Autodesk Fusion 360 part; units mm, degrees
note: some values were not read from the file. Chosen so that the rebuilt part matches the saved one: which bodies a step acts on. Set by a fixed rule: which sketch regions a step uses.
(part 3 of 6)
  spline S61 degree 5 poles (-154.2027, 37.7428) (-154.1706, 37.7034) (-154.1065, 37.6251) (-154.0104, 37.5085) (-153.8824, 37.355) (-153.7229, 37.1664) (-153.5638, 36.9811) (-153.4052, 36.7992) (-153.247, 36.6207) (-153.0893, 36.4456) (-152.9323, 36.2741) (-152.776, 36.106) (-152.6205, 35.9416) (-152.4659, 35.7807) (-152.3123, 35.6233) (-152.1597, 35.4696) (-152.0083, 35.3195) (-151.858, 35.173) (-151.709, 35.0302) (-151.5613, 34.8912) (-151.4153, 34.756) (-151.2709, 34.6246) (-151.1283, 34.4971) (-150.9877, 34.3737) (-150.8492, 34.2541) (-150.7127, 34.1386) (-150.6052, 34.0492) (-150.5255, 33.9839) (-150.4728, 33.9412) (-150.4466, 33.92) knots 0 0 0 0 0 0 0.04 0.08 0.12 0.16 0.2 0.24 0.28 0.32 0.36 0.4 0.44 0.48 0.52 0.56 0.6 0.64 0.68 0.72 0.76 0.8 0.84 0.88 0.92 0.96 1 1 1 1 1 1
  arc A61 (-156.6092, 32.582) -> (-150.4466, 33.92) centre (-153.9133, 35.0261) ccw
  spline S62 degree 5 poles (-156.6092, 32.582) (-156.5585, 32.5827) (-156.4572, 32.5839) (-156.3061, 32.5852) (-156.1063, 32.5859) (-155.8593, 32.585) (-155.6151, 32.5822) (-155.3737, 32.5776) (-155.1353, 32.5711) (-154.8999, 32.5629) (-154.6675, 32.5529) (-154.4384, 32.5411) (-154.2124, 32.5278) (-153.9898, 32.5128) (-153.7705, 32.4962) (-153.5547, 32.4782) (-153.3423, 32.4586) (-153.1335, 32.4376) (-152.9283, 32.4153) (-152.7269, 32.3915) (-152.5294, 32.3666) (-152.336, 32.3404) (-152.1468, 32.3131) (-151.9618, 32.2848) (-151.7812, 32.2555) (-151.6049, 32.2253) (-151.4674, 32.2003) (-151.3661, 32.1812) (-151.2995, 32.1683) (-151.2664, 32.1618) knots 0 0 0 0 0 0 0.04 0.08 0.12 0.16 0.2 0.24 0.28 0.32 0.36 0.4 0.44 0.48 0.52 0.56 0.6 0.64 0.68 0.72 0.76 0.8 0.84 0.88 0.92 0.96 1 1 1 1 1 1
  arc A62 (-151.2664, 32.1618) -> (-157.2099, 31.1319) centre (-153.9947, 30.2418) ccw
  spline S63 degree 5 poles (-157.2099, 31.1319) (-157.1745, 31.0955) (-157.1037, 31.0231) (-156.9978, 30.9153) (-156.857, 30.7736) (-156.6816, 30.5996) (-156.507, 30.4288) (-156.3331, 30.2614) (-156.1599, 30.0974) (-155.9876, 29.9368) (-155.8163, 29.7796) (-155.6459, 29.6258) (-155.4767, 29.4755) (-155.3087, 29.3287) (-155.1419, 29.1853) (-154.9765, 29.0455) (-154.8125, 28.9091) (-154.6501, 28.7763) (-154.4892, 28.6471) (-154.33, 28.5214) (-154.1727, 28.3994) (-154.0174, 28.2812) (-153.8643, 28.1666) (-153.7135, 28.0559) (-153.5651, 27.9489) (-153.419, 27.8456) (-153.3042, 27.766) (-153.2191, 27.7079) (-153.1628, 27.6699) (-153.1348, 27.6511) knots 0 0 0 0 0 0 0.04 0.08 0.12 0.16 0.2 0.24 0.28 0.32 0.36 0.4 0.44 0.48 0.52 0.56 0.6 0.64 0.68 0.72 0.76 0.8 0.84 0.88 0.92 0.96 1 1 1 1 1 1
  arc A63 (-159.1574, 25.7811) -> (-153.1348, 27.6511) centre (-156.6848, 28.4509) ccw
  spline S64 degree 5 poles (-159.1574, 25.7811) (-159.1069, 25.7862) (-159.0061, 25.7963) (-158.8557, 25.8107) (-158.6567, 25.8288) (-158.4106, 25.8494) (-158.167, 25.8679) (-157.9262, 25.8843) (-157.6881, 25.8987) (-157.4529, 25.911) (-157.2206, 25.9213) (-156.9913, 25.9296) (-156.765, 25.9359) (-156.5419, 25.9404) (-156.322, 25.943) (-156.1054, 25.9439) (-155.8922, 25.9429) (-155.6823, 25.9402) (-155.476, 25.9358) (-155.2733, 25.9297) (-155.0744, 25.922) (-154.8794, 25.9128) (-154.6885, 25.9021) (-154.5018, 25.8901) (-154.3193, 25.8766) (-154.1411, 25.8619) (-154.0019, 25.849) (-153.8994, 25.8388) (-153.8319, 25.8318) (-153.7983, 25.8282) knots 0 0 0 0 0 0 0.04 0.08 0.12 0.16 0.2 0.24 0.28 0.32 0.36 0.4 0.44 0.48 0.52 0.56 0.6 0.64 0.68 0.72 0.76 0.8 0.84 0.88 0.92 0.96 1 1 1 1 1 1
  arc A64 (-153.7983, 25.8282) -> (-159.6294, 24.2842) centre (-156.3488, 23.6776) ccw
  spline S65 degree 5 poles (-159.6294, 24.2842) (-159.591, 24.251) (-159.5142, 24.185) (-159.3993, 24.0869) (-159.2466, 23.9579) (-159.0568, 23.7999) (-158.8679, 23.645) (-158.6801, 23.4934) (-158.4933, 23.3451) (-158.3077, 23.2001) (-158.1232, 23.0584) (-157.9401, 22.9201) (-157.7584, 22.7851) (-157.5783, 22.6535) (-157.3997, 22.5252) (-157.2227, 22.4003) (-157.0475, 22.2788) (-156.874, 22.1606) (-156.7025, 22.0459) (-156.533, 21.9346) (-156.3656, 21.8268) (-156.2006, 21.7225) (-156.0381, 21.6218) (-155.8782, 21.5246) (-155.721, 21.4309) (-155.5666, 21.3408) (-155.4452, 21.2715) (-155.3553, 21.221) (-155.296, 21.1881) (-155.2665, 21.1718) knots 0 0 0 0 0 0 0.04 0.08 0.12 0.16 0.2 0.24 0.28 0.32 0.36 0.4 0.44 0.48 0.52 0.56 0.6 0.64 0.68 0.72 0.76 0.8 0.84 0.88 0.92 0.96 1 1 1 1 1 1
  arc A65 (-161.1032, 18.784) -> (-155.2665, 21.1718) centre (-158.8726, 21.6591) ccw
  spline S66 degree 5 poles (-161.1032, 18.784) (-161.0533, 18.7935) (-160.9538, 18.8123) (-160.8052, 18.8398) (-160.6086, 18.8751) (-160.3651, 18.9171) (-160.1241, 18.9568) (-159.8857, 18.9941) (-159.6497, 19.0292) (-159.4165, 19.062) (-159.1859, 19.0924) (-158.9582, 19.1207) (-158.7334, 19.1467) (-158.5115, 19.1706) (-158.2927, 19.1924) (-158.077, 19.2121) (-157.8644, 19.2297) (-157.6552, 19.2453) (-157.4492, 19.2589) (-157.2468, 19.2705) (-157.048, 19.2802) (-156.8529, 19.2881) (-156.6618, 19.2941) (-156.4747, 19.2983) (-156.2918, 19.3008) (-156.113, 19.3016) (-155.9732, 19.301) (-155.8702, 19.2997) (-155.8023, 19.2986) (-155.7686, 19.2979) knots 0 0 0 0 0 0 0.04 0.08 0.12 0.16 0.2 0.24 0.28 0.32 0.36 0.4 0.44 0.48 0.52 0.56 0.6 0.64 0.68 0.72 0.76 0.8 0.84 0.88 0.92 0.96 1 1 1 1 1 1
  arc A66 (-155.7686, 19.2979) -> (-161.4429, 17.2516) centre (-158.1219, 16.9333) ccw
  spline S67 degree 5 poles (-161.4429, 17.2516) (-161.4017, 17.2219) (-161.3194, 17.1628) (-161.1964, 17.0751) (-161.0331, 16.96) (-160.8302, 16.8191) (-160.6286, 16.6813) (-160.4283, 16.5466) (-160.2293, 16.4151) (-160.0317, 16.2868) (-159.8356, 16.1618) (-159.6412, 16.0399) (-159.4484, 15.9213) (-159.2574, 15.8059) (-159.0683, 15.6937) (-158.8812, 15.5847) (-158.696, 15.4789) (-158.5129, 15.3763) (-158.332, 15.277) (-158.1534, 15.1809) (-157.9773, 15.088) (-157.8039, 14.9985) (-157.6332, 14.9123) (-157.4655, 14.8294) (-157.3007, 14.7498) (-157.139, 14.6735) (-157.012, 14.615) (-156.9181, 14.5726) (-156.8561, 14.545) (-156.8253, 14.5313) knots 0 0 0 0 0 0 0.04 0.08 0.12 0.16 0.2 0.24 0.28 0.32 0.36 0.4 0.44 0.48 0.52 0.56 0.6 0.64 0.68 0.72 0.76 0.8 0.84 0.88 0.92 0.96 1 1 1 1 1 1
  arc A67 (-162.4317, 11.6439) -> (-156.8253, 14.5313) centre (-160.4602, 14.7025) ccw
  spline S68 degree 5 poles (-162.4317, 11.6439) (-162.3828, 11.6577) (-162.2853, 11.6851) (-162.1397, 11.7255) (-161.9469, 11.7778) (-161.708, 11.8408) (-161.4714, 11.9013) (-161.2371, 11.9594) (-161.0051, 12.0149) (-160.7756, 12.0678) (-160.5486, 12.1183) (-160.3242, 12.1663) (-160.1025, 12.2118) (-159.8836, 12.255) (-159.6675, 12.2957) (-159.4543, 12.3341) (-159.2441, 12.3702) (-159.037, 12.404) (-158.8331, 12.4355) (-158.6324, 12.4647) (-158.4351, 12.4917) (-158.2415, 12.5165) (-158.0517, 12.5391) (-157.8657, 12.5596) (-157.6836, 12.5781) (-157.5056, 12.5945) (-157.3663, 12.606) (-157.2635, 12.6138) (-157.1958, 12.6186) (-157.1622, 12.6208) knots 0 0 0 0 0 0 0.04 0.08 0.12 0.16 0.2 0.24 0.28 0.32 0.36 0.4 0.44 0.48 0.52 0.56 0.6 0.64 0.68 0.72 0.76 0.8 0.84 0.88 0.92 0.96 1 1 1 1 1 1
  arc A68 (-157.1622, 12.6208) -> (-162.6366, 10.0878) centre (-159.3005, 10.0601) ccw
  spline S69 degree 5 poles (-162.6366, 10.0878) (-162.5929, 10.0618) (-162.5058, 10.0101) (-162.3757, 9.9334) (-162.2029, 9.8329) (-161.9885, 9.7102) (-161.7757, 9.5905) (-161.5643, 9.4739) (-161.3546, 9.3602) (-161.1466, 9.2496) (-160.9404, 9.1422) (-160.7361, 9.0377) (-160.5337, 8.9363) (-160.3334, 8.838) (-160.1352, 8.7427) (-159.9393, 8.6504) (-159.7456, 8.5612) (-159.5543, 8.4749) (-159.3654, 8.3917) (-159.1791, 8.3116) (-158.9956, 8.2345) (-158.815, 8.1604) (-158.6375, 8.0894) (-158.4631, 8.0214) (-158.2921, 7.9565) (-158.1243, 7.8946) (-157.9927, 7.8474) (-157.8955, 7.8133) (-157.8314, 7.7912) (-157.7994, 7.7802) knots 0 0 0 0 0 0 0.04 0.08 0.12 0.16 0.2 0.24 0.28 0.32 0.36 0.4 0.44 0.48 0.52 0.56 0.6 0.64 0.68 0.72 0.76 0.8 0.84 0.88 0.92 0.96 1 1 1 1 1 1
  arc A69 (-163.1328, 4.4152) -> (-157.7994, 7.7802) centre (-161.4354, 7.634) ccw
  spline S70 degree 5 poles (-163.1328, 4.4152) (-163.0854, 4.4332) (-162.9906, 4.469) (-162.8491, 4.5219) (-162.6616, 4.5909) (-162.4291, 4.6744) (-162.1987, 4.7554) (-161.9703, 4.8336) (-161.7441, 4.9091) (-161.52, 4.9818) (-161.2983, 5.0519) (-161.0789, 5.1193) (-160.862, 5.184) (-160.6477, 5.246) (-160.436, 5.3055) (-160.227, 5.3623) (-160.0207, 5.4166) (-159.8173, 5.4683) (-159.6169, 5.5174) (-159.4195, 5.564) (-159.2254, 5.6081) (-159.0347, 5.6497) (-158.8475, 5.6888) (-158.664, 5.7254) (-158.4843, 5.7596) (-158.3083, 5.7915) (-158.1705, 5.8151) (-158.0689, 5.8318) (-158.0018, 5.8425) (-157.9685, 5.8477) knots 0 0 0 0 0 0 0.04 0.08 0.12 0.16 0.2 0.24 0.28 0.32 0.36 0.4 0.44 0.48 0.52 0.56 0.6 0.64 0.68 0.72 0.76 0.8 0.84 0.88 0.92 0.96 1 1 1 1 1 1
  arc A70 (-157.9685, 5.8477) -> (-163.2013, 2.8471) centre (-159.8755, 3.1103) ccw
  spline S71 degree 5 poles (-163.2013, 2.8471) (-163.1556, 2.825) (-163.0643, 2.7811) (-162.9279, 2.7161) (-162.7471, 2.631) (-162.5228, 2.5275) (-162.3003, 2.4268) (-162.0797, 2.329) (-161.8609, 2.2341) (-161.644, 2.1421) (-161.4292, 2.0529) (-161.2166, 1.9667) (-161.0061, 1.8834) (-160.798, 1.8029) (-160.5923, 1.7252) (-160.389, 1.6503) (-160.1883, 1.5783) (-159.9902, 1.5091) (-159.7948, 1.4426) (-159.6022, 1.379) (-159.4127, 1.3182) (-159.2263, 1.2602) (-159.0433, 1.2049) (-158.8637, 1.1524) (-158.6876, 1.1026) (-158.5151, 1.0555) (-158.3799, 1.02) (-158.2801, 0.9945) (-158.2142, 0.9781) (-158.1815, 0.97) knots 0 0 0 0 0 0 0.04 0.08 0.12 0.16 0.2 0.24 0.28 0.32 0.36 0.4 0.44 0.48 0.52 0.56 0.6 0.64 0.68 0.72 0.76 0.8 0.84 0.88 0.92 0.96 1 1 1 1 1 1
  arc A71 (-163.2013, -2.8471) -> (-158.1815, 0.97) centre (-161.7909, 0.5074) ccw
  spline S72 degree 5 poles (-163.2013, -2.8471) (-163.1556, -2.825) (-163.0643, -2.7811) (-162.9279, -2.7161) (-162.7471, -2.631) (-162.5228, -2.5275) (-162.3003, -2.4268) (-162.0797, -2.329) (-161.8609, -2.2341) (-161.644, -2.1421) (-161.4292, -2.0529) (-161.2166, -1.9667) (-161.0061, -1.8834) (-160.798, -1.8029) (-160.5923, -1.7252) (-160.389, -1.6503) (-160.1883, -1.5783) (-159.9902, -1.5091) (-159.7948, -1.4426) (-159.6022, -1.379) (-159.4127, -1.3182) (-159.2263, -1.2602) (-159.0433, -1.2049) (-158.8637, -1.1524) (-158.6876, -1.1026) (-158.5151, -1.0555) (-158.3799, -1.02) (-158.2801, -0.9945) (-158.2142, -0.9781) (-158.1815, -0.97) knots 0 0 0 0 0 0 0.04 0.08 0.12 0.16 0.2 0.24 0.28 0.32 0.36 0.4 0.44 0.48 0.52 0.56 0.6 0.64 0.68 0.72 0.76 0.8 0.84 0.88 0.92 0.96 1 1 1 1 1 1
  arc A72 (-158.1815, -0.97) -> (-163.1328, -4.4152) centre (-159.8427, -3.8631) ccw
  spline S73 degree 5 poles (-163.1328, -4.4152) (-163.0854, -4.4332) (-162.9906, -4.469) (-162.8491, -4.5219) (-162.6616, -4.5909) (-162.4291, -4.6744) (-162.1987, -4.7554) (-161.9703, -4.8336) (-161.7441, -4.9091) (-161.52, -4.9818) (-161.2983, -5.0519) (-161.0789, -5.1193) (-160.862, -5.184) (-160.6477, -5.246) (-160.436, -5.3055) (-160.227, -5.3623) (-160.0207, -5.4166) (-159.8173, -5.4683) (-159.6169, -5.5174) (-159.4195, -5.564) (-159.2254, -5.6081) (-159.0347, -5.6497) (-158.8475, -5.6888) (-158.664, -5.7254) (-158.4843, -5.7596) (-158.3083, -5.7915) (-158.1705, -5.8151) (-158.0689, -5.8318) (-158.0018, -5.8425) (-157.9685, -5.8477) knots 0 0 0 0 0 0 0.04 0.08 0.12 0.16 0.2 0.24 0.28 0.32 0.36 0.4 0.44 0.48 0.52 0.56 0.6 0.64 0.68 0.72 0.76 0.8 0.84 0.88 0.92 0.96 1 1 1 1 1 1
  arc A73 (-162.6366, -10.0878) -> (-157.9685, -5.8477) centre (-161.5239, -6.6231) ccw
  spline S74 degree 5 poles (-162.6366, -10.0878) (-162.5929, -10.0618) (-162.5058, -10.0101) (-162.3757, -9.9334) (-162.2029, -9.8329) (-161.9885, -9.7102) (-161.7757, -9.5905) (-161.5643, -9.4739) (-161.3546, -9.3602) (-161.1466, -9.2496) (-160.9404, -9.1422) (-160.7361, -9.0377) (-160.5337, -8.9363) (-160.3334, -8.838) (-160.1352, -8.7427) (-159.9393, -8.6504) (-159.7456, -8.5612) (-159.5543, -8.4749) (-159.3654, -8.3917) (-159.1791, -8.3116) (-158.9956, -8.2345) (-158.815, -8.1604) (-158.6375, -8.0894) (-158.4631, -8.0214) (-158.2921, -7.9565) (-158.1243, -7.8946) (-157.9927, -7.8474) (-157.8955, -7.8133) (-157.8314, -7.7912) (-157.7994, -7.7802) knots 0 0 0 0 0 0 0.04 0.08 0.12 0.16 0.2 0.24 0.28 0.32 0.36 0.4 0.44 0.48 0.52 0.56 0.6 0.64 0.68 0.72 0.76 0.8 0.84 0.88 0.92 0.96 1 1 1 1 1 1
  arc A74 (-157.7994, -7.7802) -> (-162.4317, -11.6439) centre (-159.2021, -10.8072) ccw
  spline S75 degree 5 poles (-162.4317, -11.6439) (-162.3828, -11.6577) (-162.2853, -11.6851) (-162.1397, -11.7255) (-161.9469, -11.7778) (-161.708, -11.8408) (-161.4714, -11.9013) (-161.2371, -11.9594) (-161.0051, -12.0149) (-160.7756, -12.0678) (-160.5486, -12.1183) (-160.3242, -12.1663) (-160.1025, -12.2118) (-159.8836, -12.255) (-159.6675, -12.2957) (-159.4543, -12.3341) (-159.2441, -12.3702) (-159.037, -12.404) (-158.8331, -12.4355) (-158.6324, -12.4647) (-158.4351, -12.4917) (-158.2415, -12.5165) (-158.0517, -12.5391) (-157.8657, -12.5596) (-157.6836, -12.5781) (-157.5056, -12.5945) (-157.3663, -12.606) (-157.2635, -12.6138) (-157.1958, -12.6186) (-157.1622, -12.6208) knots 0 0 0 0 0 0 0.04 0.08 0.12 0.16 0.2 0.24 0.28 0.32 0.36 0.4 0.44 0.48 0.52 0.56 0.6 0.64 0.68 0.72 0.76 0.8 0.84 0.88 0.92 0.96 1 1 1 1 1 1
  arc A75 (-161.4429, -17.2516) -> (-157.1622, -12.6208) centre (-160.6364, -13.7032) ccw
  spline S76 degree 5 poles (-161.4429, -17.2516) (-161.4017, -17.2219) (-161.3194, -17.1628) (-161.1964, -17.0751) (-161.0331, -16.96) (-160.8302, -16.8191) (-160.6286, -16.6813) (-160.4283, -16.5466) (-160.2293, -16.4151) (-160.0317, -16.2868) (-159.8356, -16.1618) (-159.6412, -16.0399) (-159.4484, -15.9213) (-159.2574, -15.8059) (-159.0683, -15.6937) (-158.8812, -15.5847) (-158.696, -15.4789) (-158.5129, -15.3763) (-158.332, -15.277) (-158.1534, -15.1809) (-157.9773, -15.088) (-157.8039, -14.9985) (-157.6332, -14.9123) (-157.4655, -14.8294) (-157.3007, -14.7498) (-157.139, -14.6735) (-157.012, -14.615) (-156.9181, -14.5726) (-156.8561, -14.545) (-156.8253, -14.5313) knots 0 0 0 0 0 0 0.04 0.08 0.12 0.16 0.2 0.24 0.28 0.32 0.36 0.4 0.44 0.48 0.52 0.56 0.6 0.64 0.68 0.72 0.76 0.8 0.84 0.88 0.92 0.96 1 1 1 1 1 1
  arc A76 (-156.8253, -14.5313) -> (-161.1032, -18.784) centre (-157.9589, -17.669) ccw
  spline S77 degree 5 poles (-161.1032, -18.784) (-161.0533, -18.7935) (-160.9538, -18.8123) (-160.8052, -18.8398) (-160.6086, -18.8751) (-160.3651, -18.9171) (-160.1241, -18.9568) (-159.8857, -18.9941) (-159.6497, -19.0292) (-159.4165, -19.062) (-159.1859, -19.0924) (-158.9582, -19.1207) (-158.7334, -19.1467) (-158.5115, -19.1706) (-158.2927, -19.1924) (-158.077, -19.2121) (-157.8644, -19.2297) (-157.6552, -19.2453) (-157.4492, -19.2589) (-157.2468, -19.2705) (-157.048, -19.2802) (-156.8529, -19.2881) (-156.6618, -19.2941) (-156.4747, -19.2983) (-156.2918, -19.3008) (-156.113, -19.3016) (-155.9732, -19.301) (-155.8702, -19.2997) (-155.8023, -19.2986) (-155.7686, -19.2979) knots 0 0 0 0 0 0 0.04 0.08 0.12 0.16 0.2 0.24 0.28 0.32 0.36 0.4 0.44 0.48 0.52 0.56 0.6 0.64 0.68 0.72 0.76 0.8 0.84 0.88 0.92 0.96 1 1 1 1 1 1
  arc A77 (-159.6294, -24.2842) -> (-155.7686, -19.2979) centre (-159.1352, -20.679) ccw
  spline S78 degree 5 poles (-159.6294, -24.2842) (-159.591, -24.251) (-159.5142, -24.185) (-159.3993, -24.0869) (-159.2466, -23.9579) (-159.0568, -23.7999) (-158.8679, -23.645) (-158.6801, -23.4934) (-158.4933, -23.3451) (-158.3077, -23.2001) (-158.1232, -23.0584) (-157.9401, -22.9201) (-157.7584, -22.7851) (-157.5783, -22.6535) (-157.3997, -22.5252) (-157.2227, -22.4003) (-157.0475, -22.2788) (-156.874, -22.1606) (-156.7025, -22.0459) (-156.533, -21.9346) (-156.3656, -21.8268) (-156.2006, -21.7225) (-156.0381, -21.6218) (-155.8782, -21.5246) (-155.721, -21.4309) (-155.5666, -21.3408) (-155.4452, -21.2715) (-155.3553, -21.221) (-155.296, -21.1881) (-155.2665, -21.1718) knots 0 0 0 0 0 0 0.04 0.08 0.12 0.16 0.2 0.24 0.28 0.32 0.36 0.4 0.44 0.48 0.52 0.56 0.6 0.64 0.68 0.72 0.76 0.8 0.84 0.88 0.92 0.96 1 1 1 1 1 1
  arc A78 (-155.2665, -21.1718) -> (-159.1574, -25.7811) centre (-156.1222, -24.3963) ccw
  spline S79 degree 5 poles (-159.1574, -25.7811) (-159.1069, -25.7862) (-159.0061, -25.7963) (-158.8557, -25.8107) (-158.6567, -25.8288) (-158.4106, -25.8494) (-158.167, -25.8679) (-157.9262, -25.8843) (-157.6881, -25.8987) (-157.4529, -25.911) (-157.2206, -25.9213) (-156.9913, -25.9296) (-156.765, -25.9359) (-156.5419, -25.9404) (-156.322, -25.943) (-156.1054, -25.9439) (-155.8922, -25.9429) (-155.6823, -25.9402) (-155.476, -25.9358) (-155.2733, -25.9297) (-155.0744, -25.922) (-154.8794, -25.9128) (-154.6885, -25.9021) (-154.5018, -25.8901) (-154.3193, -25.8766) (-154.1411, -25.8619) (-154.0019, -25.849) (-153.8994, -25.8388) (-153.8319, -25.8318) (-153.7983, -25.8282) knots 0 0 0 0 0 0 0.04 0.08 0.12 0.16 0.2 0.24 0.28 0.32 0.36 0.4 0.44 0.48 0.52 0.56 0.6 0.64 0.68 0.72 0.76 0.8 0.84 0.88 0.92 0.96 1 1 1 1 1 1
  arc A79 (-157.2099, -31.1319) -> (-153.7983, -25.8282) centre (-157.0318, -27.4974) ccw
  spline S80 degree 5 poles (-157.2099, -31.1319) (-157.1745, -31.0955) (-157.1037, -31.0231) (-156.9978, -30.9153) (-156.857, -30.7736) (-156.6816, -30.5996) (-156.507, -30.4288) (-156.3331, -30.2614) (-156.1599, -30.0974) (-155.9876, -29.9368) (-155.8163, -29.7796) (-155.6459, -29.6258) (-155.4767, -29.4755) (-155.3087, -29.3287) (-155.1419, -29.1853) (-154.9765, -29.0455) (-154.8125, -28.9091) (-154.6501, -28.7763) (-154.4892, -28.6471) (-154.33, -28.5214) (-154.1727, -28.3994) (-154.0174, -28.2812) (-153.8643, -28.1666) (-153.7135, -28.0559) (-153.5651, -27.9489) (-153.419, -27.8456) (-153.3042, -27.766) (-153.2191, -27.7079) (-153.1628, -27.6699) (-153.1348, -27.6511) knots 0 0 0 0 0 0 0.04 0.08 0.12 0.16 0.2 0.24 0.28 0.32 0.36 0.4 0.44 0.48 0.52 0.56 0.6 0.64 0.68 0.72 0.76 0.8 0.84 0.88 0.92 0.96 1 1 1 1 1 1
  arc A80 (-153.1348, -27.6511) -> (-156.6092, -32.582) centre (-153.7063, -30.938) ccw
  spline S81 degree 5 poles (-156.6092, -32.582) (-156.5585, -32.5827) (-156.4572, -32.5839) (-156.3061, -32.5852) (-156.1063, -32.5859) (-155.8593, -32.585) (-155.6151, -32.5822) (-155.3737, -32.5776) (-155.1353, -32.5711) (-154.8999, -32.5629) (-154.6675, -32.5529) (-154.4384, -32.5411) (-154.2124, -32.5278) (-153.9898, -32.5128) (-153.7705, -32.4962) (-153.5547, -32.4782) (-153.3423, -32.4586) (-153.1335, -32.4376) (-152.9283, -32.4153) (-152.7269, -32.3915) (-152.5294, -32.3666) (-152.336, -32.3404) (-152.1468, -32.3131) (-151.9618, -32.2848) (-151.7812, -32.2555) (-151.6049, -32.2253) (-151.4674, -32.2003) (-151.3661, -32.1812) (-151.2995, -32.1683) (-151.2664, -32.1618) knots 0 0 0 0 0 0 0.04 0.08 0.12 0.16 0.2 0.24 0.28 0.32 0.36 0.4 0.44 0.48 0.52 0.56 0.6 0.64 0.68 0.72 0.76 0.8 0.84 0.88 0.92 0.96 1 1 1 1 1 1
  arc A81 (-154.2027, -37.7428) -> (-151.2664, -32.1618) centre (-154.3421, -34.1065) ccw
  spline S82 degree 5 poles (-154.2027, -37.7428) (-154.1706, -37.7034) (-154.1065, -37.6251) (-154.0104, -37.5085) (-153.8824, -37.355) (-153.7229, -37.1664) (-153.5638, -36.9811) (-153.4052, -36.7992) (-153.247, -36.6207) (-153.0893, -36.4456) (-152.9323, -36.2741) (-152.776, -36.106) (-152.6205, -35.9416) (-152.4659, -35.7807) (-152.3123, -35.6233) (-152.1597, -35.4696) (-152.0083, -35.3195) (-151.858, -35.173) (-151.709, -35.0302) (-151.5613, -34.8912) (-151.4153, -34.756) (-151.2709, -34.6246) (-151.1283, -34.4971) (-150.9877, -34.3737) (-150.8492, -34.2541) (-150.7127, -34.1386) (-150.6052, -34.0492) (-150.5255, -33.9839) (-150.4728, -33.9412) (-150.4466, -33.92) knots 0 0 0 0 0 0 0.04 0.08 0.12 0.16 0.2 0.24 0.28 0.32 0.36 0.4 0.44 0.48 0.52 0.56 0.6 0.64 0.68 0.72 0.76 0.8 0.84 0.88 0.92 0.96 1 1 1 1 1 1
  arc A82 (-150.4466, -33.92) -> (-153.478, -39.135) centre (-150.7294, -37.2442) ccw
  spline S83 degree 5 poles (-153.478, -39.135) (-153.4274, -39.1312) (-153.3264, -39.1236) (-153.1757, -39.1118) (-152.9766, -39.095) (-152.7306, -39.0725) (-152.4876, -39.0485) (-152.2476, -39.0229) (-152.0106, -38.9957) (-151.7768, -38.9669) (-151.5462, -38.9367) (-151.319, -38.905) (-151.095, -38.872) (-150.8746, -38.8377) (-150.6576, -38.8021) (-150.4441, -38.7653) (-150.2343, -38.7273) (-150.0281, -38.6882) (-149.8256, -38.648) (-149.6271, -38.6069) (-149.4325, -38.5648) (-149.2421, -38.5218) (-149.0559, -38.4782) (-148.8742, -38.4338) (-148.6968, -38.3889) (-148.5238, -38.3434) (-148.389, -38.3066) (-148.2898, -38.2788) (-148.2245, -38.2601) (-148.1921, -38.2507) knots 0 0 0 0 0 0 0.04 0.08 0.12 0.16 0.2 0.24 0.28 0.32 0.36 0.4 0.44 0.48 0.52 0.56 0.6 0.64 0.68 0.72 0.76 0.8 0.84 0.88 0.92 0.96 1 1 1 1 1 1
  arc A83 (-150.6309, -44.0663) -> (-148.1921, -38.2507) centre (-151.0867, -40.4561) ccw
  spline S84 degree 5 poles (-150.6309, -44.0663) (-150.6023, -44.0243) (-150.5452, -43.9407) (-150.4597, -43.8162) (-150.3456, -43.6521) (-150.2031, -43.4503) (-150.0608, -43.2519) (-149.9186, -43.0568) (-149.7765, -42.8652) (-149.6348, -42.6771) (-149.4933, -42.4925) (-149.3522, -42.3115) (-149.2117, -42.1341) (-149.0717, -41.9603) (-148.9324, -41.7902) (-148.7938, -41.6237) (-148.656, -41.461) (-148.519, -41.302) (-148.383, -41.1468) (-148.2481, -40.9954) (-148.1143, -40.8479) (-147.9819, -40.7045) (-147.851, -40.5651) (-147.7217, -40.4299) (-147.5942, -40.2987) (-147.4683, -40.1717) (-147.369, -40.0733) (-147.2953, -40.0013) (-147.2465, -39.9541) (-147.2222, -39.9308) knots 0 0 0 0 0 0 0.04 0.08 0.12 0.16 0.2 0.24 0.28 0.32 0.36 0.4 0.44 0.48 0.52 0.56 0.6 0.64 0.68 0.72 0.76 0.8 0.84 0.88 0.92 0.96 1 1 1 1 1 1
  arc A84 (-147.2222, -39.9308) -> (-149.7876, -45.3901) centre (-147.2142, -43.2669) ccw
  spline S85 degree 5 poles (-149.7876, -45.3901) (-149.7374, -45.3819) (-149.6375, -45.3656) (-149.4885, -45.3406) (-149.2916, -45.3066) (-149.0485, -45.2627) (-148.8085, -45.2176) (-148.5716, -45.1711) (-148.3379, -45.1234) (-148.1075, -45.0744) (-147.8804, -45.0242) (-147.6568, -44.9729) (-147.4366, -44.9204) (-147.2199, -44.867) (-147.0069, -44.8126) (-146.7974, -44.7574) (-146.5917, -44.7013) (-146.3897, -44.6443) (-146.1915, -44.5867) (-145.9973, -44.5283) (-145.8072, -44.4694) (-145.6212, -44.4101) (-145.4396, -44.3504) (-145.2623, -44.2904) (-145.0896, -44.2301) (-144.9212, -44.1698) (-144.7901, -44.1213) (-144.6937, -44.0849) (-144.6303, -44.0607) (-144.5989, -44.0485) knots 0 0 0 0 0 0 0.04 0.08 0.12 0.16 0.2 0.24 0.28 0.32 0.36 0.4 0.44 0.48 0.52 0.56 0.6 0.64 0.68 0.72 0.76 0.8 0.84 0.88 0.92 0.96 1 1 1 1 1 1
  arc A85 (-146.5215, -50.0545) -> (-144.5989, -44.0485) centre (-147.2902, -46.4977) ccw
  spline S86 degree 5 poles (-146.5215, -50.0545) (-146.4967, -50.0102) (-146.4471, -49.9219) (-146.3727, -49.7904) (-146.2734, -49.617) (-146.149, -49.4036) (-146.0245, -49.1935) (-145.8999, -48.9868) (-145.7751, -48.7835) (-145.6502, -48.5838) (-145.5254, -48.3875) (-145.4006, -48.1949) (-145.2761, -48.006) (-145.1518, -47.8206) (-145.0278, -47.639) (-144.9042, -47.4611) (-144.7811, -47.287) (-144.6586, -47.1166) (-144.5366, -46.9502) (-144.4154, -46.7876) (-144.295, -46.6291) (-144.1756, -46.4746) (-144.0574, -46.3244) (-143.9404, -46.1783) (-143.8247, -46.0366) (-143.7104, -45.8991) (-143.62, -45.7924) (-143.5529, -45.7143) (-143.5084, -45.663) (-143.4862, -45.6376) knots 0 0 0 0 0 0 0.04 0.08 0.12 0.16 0.2 0.24 0.28 0.32 0.36 0.4 0.44 0.48 0.52 0.56 0.6 0.64 0.68 0.72 0.76 0.8 0.84 0.88 0.92 0.96 1 1 1 1 1 1
  arc A86 (-143.4862, -45.6376) -> (-145.566, -51.2997) centre (-143.1875, -48.9604) ccw
  spline S87 degree 5 poles (-145.566, -51.2997) (-145.5168, -51.2873) (-145.4186, -51.2622) (-145.2724, -51.2244) (-145.0792, -51.1733) (-144.8408, -51.1085) (-144.6057, -51.0426) (-144.3737, -50.9757) (-144.1451, -50.9077) (-143.9198, -50.8388) (-143.698, -50.769) (-143.4797, -50.6984) (-143.2649, -50.627) (-143.0537, -50.5549) (-142.8462, -50.4821) (-142.6424, -50.4088) (-142.4423, -50.335) (-142.2461, -50.2607) (-142.0537, -50.186) (-141.8653, -50.1109) (-141.681, -50.0357) (-141.5009, -49.9604) (-141.3252, -49.885) (-141.1538, -49.8098) (-140.987, -49.7348) (-140.8245, -49.6599) (-140.6981, -49.6003) (-140.6053, -49.5556) (-140.5443, -49.5259) (-140.514, -49.511) knots 0 0 0 0 0 0 0.04 0.08 0.12 0.16 0.2 0.24 0.28 0.32 0.36 0.4 0.44 0.48 0.52 0.56 0.6 0.64 0.68 0.72 0.76 0.8 0.84 0.88 0.92 0.96 1 1 1 1 1 1
  arc A87 (-141.9058, -55.6618) -> (-140.514, -49.511) centre (-142.9816, -52.1855) ccw
  spline S88 degree 5 poles (-141.9058, -55.6618) (-141.885, -55.6155) (-141.8433, -55.5232) (-141.7806, -55.3857) (-141.6968, -55.2043) (-141.5915, -54.9809) (-141.4858, -54.7607) (-141.3796, -54.5439) (-141.273, -54.3305) (-141.1661, -54.1207) (-141.0588, -53.9143) (-140.9513, -53.7116) (-140.8437, -53.5125) (-140.736, -53.317) (-140.6283, -53.1253) (-140.5207, -52.9373) (-140.4133, -52.7531) (-140.306, -52.5727) (-140.199, -52.3962) (-140.0924, -52.2237) (-139.9863, -52.0553) (-139.8809, -51.891) (-139.7762, -51.7311) (-139.6723, -51.5754) (-139.5695, -51.4241) (-139.4676, -51.2771) (-139.3868, -51.163) (-139.3268, -51.0793) (-139.2869, -51.0244) (-139.267, -50.9971) knots 0 0 0 0 0 0 0.04 0.08 0.12 0.16 0.2 0.24 0.28 0.32 0.36 0.4 0.44 0.48 0.52 0.56 0.6 0.64 0.68 0.72 0.76 0.8 0.84 0.88 0.92 0.96 1 1 1 1 1 1
  arc A88 (-139.267, -50.9971) -> (-140.8454, -56.819) centre (-138.6799, -54.2812) ccw
  spline S89 degree 5 poles (-140.8454, -56.819) (-140.7975, -56.8023) (-140.7019, -56.7688) (-140.5595, -56.7183) (-140.3715, -56.6506) (-140.1397, -56.5652) (-139.9112, -56.4791) (-139.6859, -56.3922) (-139.4641, -56.3046) (-139.2457, -56.2164) (-139.0308, -56.1275) (-138.8195, -56.0381) (-138.6117, -55.9482) (-138.4076, -55.858) (-138.2072, -55.7675) (-138.0106, -55.6767) (-137.8177, -55.5857) (-137.6287, -55.4945) (-137.4436, -55.4033) (-137.2624, -55.3122) (-137.0854, -55.2211) (-136.9125, -55.1304) (-136.744, -55.04) (-136.5799, -54.9502) (-136.4202, -54.8609) (-136.2649, -54.7722) (-136.1442, -54.7017) (-136.0556, -54.6491) (-135.9974, -54.6142) (-135.9685, -54.5968) knots 0 0 0 0 0 0 0.04 0.08 0.12 0.16 0.2 0.24 0.28 0.32 0.36 0.4 0.44 0.48 0.52 0.56 0.6 0.64 0.68 0.72 0.76 0.8 0.84 0.88 0.92 0.96 1 1 1 1 1 1
  arc A89 (-136.819, -60.8454) -> (-135.9685, -54.5968) centre (-138.1936, -57.4761) ccw
  spline S90 degree 5 poles (-136.819, -60.8454) (-136.8023, -60.7975) (-136.7688, -60.7019) (-136.7183, -60.5595) (-136.6506, -60.3715) (-136.5652, -60.1397) (-136.4791, -59.9112) (-136.3922, -59.6859) (-136.3046, -59.4641) (-136.2164, -59.2457) (-136.1275, -59.0308) (-136.0381, -58.8195) (-135.9482, -58.6117) (-135.858, -58.4076) (-135.7675, -58.2072) (-135.6767, -58.0106) (-135.5857, -57.8177) (-135.4945, -57.6287) (-135.4033, -57.4436) (-135.3122, -57.2624) (-135.2211, -57.0854) (-135.1304, -56.9125) (-135.04, -56.744) (-134.9502, -56.5799) (-134.8609, -56.4202) (-134.7722, -56.2649) (-134.7017, -56.1442) (-134.6491, -56.0556) (-134.6142, -55.9974) (-134.5968, -55.9685) knots 0 0 0 0 0 0 0.04 0.08 0.12 0.16 0.2 0.24 0.28 0.32 0.36 0.4 0.44 0.48 0.52 0.56 0.6 0.64 0.68 0.72 0.76 0.8 0.84 0.88 0.92 0.96 1 1 1 1 1 1
  arc A90 (-134.5968, -55.9685) -> (-135.6618, -61.9058) centre (-133.7256, -59.1889) ccw
  spline S91 degree 5 poles (-135.6618, -61.9058) (-135.6155, -61.885) (-135.5232, -61.8433) (-135.3857, -61.7806) (-135.2043, -61.6968) (-134.9809, -61.5915) (-134.7607, -61.4858) (-134.5439, -61.3796) (-134.3305, -61.273) (-134.1207, -61.1661) (-133.9143, -61.0588) (-133.7116, -60.9513) (-133.5125, -60.8437) (-133.317, -60.736) (-133.1253, -60.6283) (-132.9373, -60.5207) (-132.7531, -60.4133) (-132.5727, -60.306) (-132.3962, -60.199) (-132.2237, -60.0924) (-132.0553, -59.9863) (-131.891, -59.8809) (-131.7311, -59.7762) (-131.5754, -59.6723) (-131.4241, -59.5695) (-131.2771, -59.4676) (-131.163, -59.3868) (-131.0793, -59.3268) (-131.0244, -59.2869) (-130.9971, -59.267) knots 0 0 0 0 0 0 0.04 0.08 0.12 0.16 0.2 0.24 0.28 0.32 0.36 0.4 0.44 0.48 0.52 0.56 0.6 0.64 0.68 0.72 0.76 0.8 0.84 0.88 0.92 0.96 1 1 1 1 1 1
  arc A91 (-131.2997, -65.566) -> (-130.9971, -59.267) centre (-132.9628, -62.3293) ccw
  spline S92 degree 5 poles (-131.2997, -65.566) (-131.2873, -65.5168) (-131.2622, -65.4186) (-131.2244, -65.2724) (-131.1733, -65.0792) (-131.1085, -64.8408) (-131.0426, -64.6057) (-130.9757, -64.3737) (-130.9077, -64.1451) (-130.8388, -63.9198) (-130.769, -63.698) (-130.6984, -63.4797) (-130.627, -63.2649) (-130.5549, -63.0537) (-130.4821, -62.8462) (-130.4088, -62.6424) (-130.335, -62.4423) (-130.2607, -62.2461) (-130.186, -62.0537) (-130.1109, -61.8653) (-130.0357, -61.681) (-129.9604, -61.5009) (-129.885, -61.3252) (-129.8098, -61.1538) (-129.7348, -60.987) (-129.6599, -60.8245) (-129.6003, -60.6981) (-129.5556, -60.6053) (-129.5259, -60.5443) (-129.511, -60.514) knots 0 0 0 0 0 0 0.04 0.08 0.12 0.16 0.2 0.24 0.28 0.32 0.36 0.4 0.44 0.48 0.52 0.56 0.6 0.64 0.68 0.72 0.76 0.8 0.84 0.88 0.92 0.96 1 1 1 1 1 1
  arc A92 (-129.511, -60.514) -> (-130.0545, -66.5215) centre (-128.3625, -63.6462) ccw
  spline S93 degree 5 poles (-130.0545, -66.5215) (-130.0102, -66.4967) (-129.9219, -66.4471) (-129.7904, -66.3727) (-129.617, -66.2734) (-129.4036, -66.149) (-129.1935, -66.0245) (-128.9868, -65.8999) (-128.7835, -65.7751) (-128.5838, -65.6502) (-128.3875, -65.5254) (-128.1949, -65.4006) (-128.006, -65.2761) (-127.8206, -65.1518) (-127.639, -65.0278) (-127.4611, -64.9042) (-127.287, -64.7811) (-127.1166, -64.6586) (-126.9502, -64.5366) (-126.7876, -64.4154) (-126.6291, -64.295) (-126.4746, -64.1756) (-126.3244, -64.0574) (-126.1783, -63.9404) (-126.0366, -63.8247) (-125.8991, -63.7104) (-125.7924, -63.62) (-125.7143, -63.5529) (-125.663, -63.5084) (-125.6376, -63.4862) knots 0 0 0 0 0 0 0.04 0.08 0.12 0.16 0.2 0.24 0.28 0.32 0.36 0.4 0.44 0.48 0.52 0.56 0.6 0.64 0.68 0.72 0.76 0.8 0.84 0.88 0.92 0.96 1 1 1 1 1 1
  arc A93 (-125.3901, -69.7876) -> (-125.6376, -63.4862) centre (-127.3289, -66.7082) ccw
  spline S94 degree 5 poles (-125.3901, -69.7876) (-125.3819, -69.7374) (-125.3656, -69.6375) (-125.3406, -69.4885) (-125.3066, -69.2916) (-125.2627, -69.0485) (-125.2176, -68.8085) (-125.1711, -68.5716) (-125.1234, -68.3379) (-125.0744, -68.1075) (-125.0242, -67.8804) (-124.9729, -67.6568) (-124.9204, -67.4366) (-124.867, -67.2199) (-124.8126, -67.0069) (-124.7574, -66.7974) (-124.7013, -66.5917) (-124.6443, -66.3897) (-124.5867, -66.1915) (-124.5283, -65.9973) (-124.4694, -65.8072) (-124.4101, -65.6212) (-124.3504, -65.4396) (-124.2904, -65.2623) (-124.2301, -65.0896) (-124.1698, -64.9212) (-124.1213, -64.7901) (-124.0849, -64.6937) (-124.0607, -64.6303) (-124.0485, -64.5989) knots 0 0 0 0 0 0 0.04 0.08 0.12 0.16 0.2 0.24 0.28 0.32 0.36 0.4 0.44 0.48 0.52 0.56 0.6 0.64 0.68 0.72 0.76 0.8 0.84 0.88 0.92 0.96 1 1 1 1 1 1
  arc A94 (-124.0485, -64.5989) -> (-124.0663, -70.6309) centre (-122.6314, -67.6191) ccw
  spline S95 degree 5 poles (-124.0663, -70.6309) (-124.0243, -70.6023) (-123.9407, -70.5452) (-123.8162, -70.4597) (-123.6521, -70.3456) (-123.4503, -70.2031) (-123.2519, -70.0608) (-123.0568, -69.9186) (-122.8652, -69.7765) (-122.6771, -69.6348) (-122.4925, -69.4933) (-122.3115, -69.3522) (-122.1341, -69.2117) (-121.9603, -69.0717) (-121.7902, -68.9324) (-121.6237, -68.7938) (-121.461, -68.656) (-121.302, -68.519) (-121.1468, -68.383) (-120.9954, -68.2481) (-120.8479, -68.1143) (-120.7045, -67.9819) (-120.5651, -67.851) (-120.4299, -67.7217) (-120.2987, -67.5942) (-120.1717, -67.4683) (-120.0733, -67.369) (-120.0013, -67.2953) (-119.9541, -67.2465) (-119.9308, -67.2222) knots 0 0 0 0 0 0 0.04 0.08 0.12 0.16 0.2 0.24 0.28 0.32 0.36 0.4 0.44 0.48 0.52 0.56 0.6 0.64 0.68 0.72 0.76 0.8 0.84 0.88 0.92 0.96 1 1 1 1 1 1
  arc A95 (-119.135, -73.478) -> (-119.9308, -67.2222) centre (-121.3348, -70.5793) ccw
  spline S96 degree 5 poles (-119.135, -73.478) (-119.1312, -73.4274) (-119.1236, -73.3264) (-119.1118, -73.1757) (-119.095, -72.9766) (-119.0725, -72.7306) (-119.0485, -72.4876) (-119.0229, -72.2476) (-118.9957, -72.0106) (-118.9669, -71.7768) (-118.9367, -71.5462) (-118.905, -71.319) (-118.872, -71.095) (-118.8377, -70.8746) (-118.8021, -70.6576) (-118.7653, -70.4441) (-118.7273, -70.2343) (-118.6882, -70.0281) (-118.648, -69.8256) (-118.6069, -69.6271) (-118.5648, -69.4325) (-118.5218, -69.2421) (-118.4782, -69.0559) (-118.4338, -68.8742) (-118.3889, -68.6968) (-118.3434, -68.5238) (-118.3066, -68.389) (-118.2788, -68.2898) (-118.2601, -68.2245) (-118.2507, -68.1921) knots 0 0 0 0 0 0 0.04 0.08 0.12 0.16 0.2 0.24 0.28 0.32 0.36 0.4 0.44 0.48 0.52 0.56 0.6 0.64 0.68 0.72 0.76 0.8 0.84 0.88 0.92 0.96 1 1 1 1 1 1
  arc A96 (-118.2507, -68.1921) -> (-117.7428, -74.2027) centre (-116.5758, -71.0773) ccw
  spline S97 degree 5 poles (-117.7428, -74.2027) (-117.7034, -74.1706) (-117.6251, -74.1065) (-117.5085, -74.0104) (-117.355, -73.8824) (-117.1664, -73.7229) (-116.9811, -73.5638) (-116.7992, -73.4052) (-116.6207, -73.247) (-116.4456, -73.0893) (-116.2741, -72.9323) (-116.106, -72.776) (-115.9416, -72.6205) (-115.7807, -72.4659) (-115.6233, -72.3123) (-115.4696, -72.1597) (-115.3195, -72.0083) (-115.173, -71.858) (-115.0302, -71.709) (-114.8912, -71.5613) (-114.756, -71.4153) (-114.6246, -71.2709) (-114.4971, -71.1283) (-114.3737, -70.9877) (-114.2541, -70.8492) (-114.1386, -70.7127) (-114.0492, -70.6052) (-113.9839, -70.5255) (-113.9412, -70.4728) (-113.92, -70.4466) knots 0 0 0 0 0 0 0.04 0.08 0.12 0.16 0.2 0.24 0.28 0.32 0.36 0.4 0.44 0.48 0.52 0.56 0.6 0.64 0.68 0.72 0.76 0.8 0.84 0.88 0.92 0.96 1 1 1 1 1 1
  arc A97 (-112.582, -76.6092) -> (-113.92, -70.4466) centre (-115.0261, -73.9133) ccw
  spline S98 degree 5 poles (-112.582, -76.6092) (-112.5827, -76.5585) (-112.5839, -76.4572) (-112.5852, -76.3061) (-112.5859, -76.1063) (-112.585, -75.8593) (-112.5822, -75.6151) (-112.5776, -75.3737) (-112.5711, -75.1353) (-112.5629, -74.8999) (-112.5529, -74.6675) (-112.5411, -74.4384) (-112.5278, -74.2124) (-112.5128, -73.9898) (-112.4962, -73.7705) (-112.4782, -73.5547) (-112.4586, -73.3423) (-112.4376, -73.1335) (-112.4153, -72.9283) (-112.3915, -72.7269) (-112.3666, -72.5294) (-112.3404, -72.336) (-112.3131, -72.1468) (-112.2848, -71.9618) (-112.2555, -71.7812) (-112.2253, -71.6049) (-112.2003, -71.4674) (-112.1812, -71.3661) (-112.1683, -71.2995) (-112.1618, -71.2664) knots 0 0 0 0 0 0 0.04 0.08 0.12 0.16 0.2 0.24 0.28 0.32 0.36 0.4 0.44 0.48 0.52 0.56 0.6 0.64 0.68 0.72 0.76 0.8 0.84 0.88 0.92 0.96 1 1 1 1 1 1
  arc A98 (-112.1618, -71.2664) -> (-111.1319, -77.2099) centre (-110.2418, -73.9947) ccw
  spline S99 degree 5 poles (-111.1319, -77.2099) (-111.0955, -77.1745) (-111.0231, -77.1037) (-110.9153, -76.9978) (-110.7736, -76.857) (-110.5996, -76.6816) (-110.4288, -76.507) (-110.2614, -76.3331) (-110.0974, -76.1599) (-109.9368, -75.9876) (-109.7796, -75.8163) (-109.6258, -75.6459) (-109.4755, -75.4767) (-109.3287, -75.3087) (-109.1853, -75.1419) (-109.0455, -74.9765) (-108.9091, -74.8125) (-108.7763, -74.6501) (-108.6471, -74.4892) (-108.5214, -74.33) (-108.3994, -74.1727) (-108.2812, -74.0174) (-108.1666, -73.8643) (-108.0559, -73.7135) (-107.9489, -73.5651) (-107.8456, -73.419) (-107.766, -73.3042) (-107.7079, -73.2191) (-107.6699, -73.1628) (-107.6511, -73.1348) knots 0 0 0 0 0 0 0.04 0.08 0.12 0.16 0.2 0.24 0.28 0.32 0.36 0.4 0.44 0.48 0.52 0.56 0.6 0.64 0.68 0.72 0.76 0.8 0.84 0.88 0.92 0.96 1 1 1 1 1 1
  arc A99 (-105.7811, -79.1574) -> (-107.6511, -73.1348) centre (-108.4509, -76.6848) ccw
  spline S100 degree 5 poles (-105.7811, -79.1574) (-105.7862, -79.1069) (-105.7963, -79.0061) (-105.8107, -78.8557) (-105.8288, -78.6567) (-105.8494, -78.4106) (-105.8679, -78.167) (-105.8843, -77.9262) (-105.8987, -77.6881) (-105.911, -77.4529) (-105.9213, -77.2206) (-105.9296, -76.9913) (-105.9359, -76.765) (-105.9404, -76.5419) (-105.943, -76.322) (-105.9439, -76.1054) (-105.9429, -75.8922) (-105.9402, -75.6823) (-105.9358, -75.476) (-105.9297, -75.2733) (-105.922, -75.0744) (-105.9128, -74.8794) (-105.9021, -74.6885) (-105.8901, -74.5018) (-105.8766, -74.3193) (-105.8619, -74.1411) (-105.849, -74.0019) (-105.8388, -73.8994) (-105.8318, -73.8319) (-105.8282, -73.7983) knots 0 0 0 0 0 0 0.04 0.08 0.12 0.16 0.2 0.24 0.28 0.32 0.36 0.4 0.44 0.48 0.52 0.56 0.6 0.64 0.68 0.72 0.76 0.8 0.84 0.88 0.92 0.96 1 1 1 1 1 1
  arc A100 (-105.8282, -73.7983) -> (-104.2842, -79.6294) centre (-103.6776, -76.3488) ccw
  spline S101 degree 5 poles (-104.2842, -79.6294) (-104.251, -79.591) (-104.185, -79.5142) (-104.0869, -79.3993) (-103.9579, -79.2466) (-103.7999, -79.0568) (-103.645, -78.8679) (-103.4934, -78.6801) (-103.3451, -78.4933) (-103.2001, -78.3077) (-103.0584, -78.1232) (-102.9201, -77.9401) (-102.7851, -77.7584) (-102.6535, -77.5783) (-102.5252, -77.3997) (-102.4003, -77.2227) (-102.2788, -77.0475) (-102.1606, -76.874) (-102.0459, -76.7025) (-101.9346, -76.533) (-101.8268, -76.3656) (-101.7225, -76.2006) (-101.6218, -76.0381) (-101.5246, -75.8782) (-101.4309, -75.721) (-101.3408, -75.5666) (-101.2715, -75.4452) (-101.221, -75.3553) (-101.1881, -75.296) (-101.1718, -75.2665) knots 0 0 0 0 0 0 0.04 0.08 0.12 0.16 0.2 0.24 0.28 0.32 0.36 0.4 0.44 0.48 0.52 0.56 0.6 0.64 0.68 0.72 0.76 0.8 0.84 0.88 0.92 0.96 1 1 1 1 1 1
  arc A101 (-98.784, -81.1032) -> (-101.1718, -75.2665) centre (-101.6591, -78.8726) ccw